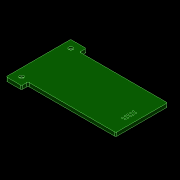
# Autodesk Inventor part: hw_DAA - PCB Peripherals
Saved by Autodesk Inventor 2018 (Build 220112000, 112)
## iProperties
Created: 2024-03-13
Part Number: hw_DAA - PCB Peripherals
Material: PCB
Document SubType Name: Modeling
Designer: cda1
Density: 4 g/cm^3
Appearance: PCB
Author: cda1
Autodesk Inventor part; units mm, degrees
ref_plane "YZ Plane" through (0, 0, 0) normal (1, 0, 0) x (0, 1, 0)
ref_plane "XZ Plane" through (0, 0, 0) normal (0, 1, 0) x (-1, 0, 0)
ref_plane "XY Plane" through (0, 0, 0) normal (0, 0, 1) x (1, 0, 0)
sketch "Boceto1" plane through (0, 0, 0) normal (0, 0, 1) x (1, 0, 0)
  line L0 (-26, 17) -> (26, 17)
  line L1 (26, 17) -> (26, -17)
  line L2 (26, -17) -> (-26, -17)
  line L3 (-26, -17) -> (-26, 17)
  line L4 (-26, 17) -> (26, -17) construction
  line L5 (26, 17) -> (-26, -17) construction
  point P0 (0, 0)
  dimension "d0" = 52
  dimension "d1" = 34
  constraints: 12 end point, 2 midpoint, 2 parallel, 1 horizontal, 1 perpendicular
  measures "d0" distance of L1.end L2.end
  measures "d1" distance of L0.end L1.end
extrude "Extrusión1" add sketch "Boceto1" against normal blind 1.742
fillet "Empalme1" radius 0.5 4 edges at (26, 17, -0.871) (-26, 17, -0.871) (-26, -17, -0.871) (26, -17, -0.871)
sketch "Boceto2" plane through (0, 0, -1.742) normal (0, 0, -1) x (-1, 0, 0)
  line L0 (-25.5, 17) -> (25.5, 17) projected
  line L1 (25.5, -17) -> (-25.5, -17) projected
  line L2 (25.5, 17) -> (-25.5, 17) projected
  line L3 (15.5, 17) -> (-26, 17)
  line L4 (-26, 17) -> (-26, 12.2)
  line L5 (-26, 12.2) -> (15.5, 12.2)
  line L6 (15.5, 12.2) -> (15.5, 17)
  line L7 (-26, -16.5) -> (-26, 16.5) projected
  line L8 (-25.5, -17) -> (25.5, -17) projected
  line L9 (-26, 16.5) -> (-26, -16.5) projected
  line L10 (15.5, -17) -> (-26, -17)
  line L11 (-26, -17) -> (-26, -12.2)
  line L12 (-26, -12.2) -> (15.5, -12.2)
  line L13 (15.5, -12.2) -> (15.5, -17)
  point P0 (0, 0)
  dimension "d5" = 4.8
  dimension "d6" = 41.5
  dimension "d7" = 4.8
  dimension "d8" = 41.5
  constraints: 16 end point, 4 parallel, 4 point on line, 2 horizontal, 2 perpendicular
  measures "d5" distance of L4.end L3.end
  measures "d6" distance of L4.end L5.end
  measures "d7" distance of L10.end L11.end
  measures "d8" distance of L11.end L12.end
extrude "Extrusión2" cut sketch "Boceto2" against normal through all
sketch "Boceto4" plane through (0, 0, 0) normal (0, 0, 1) x (1, 0, 0)
  line L0 (-26, -16.5) -> (-26, 16.5) construction
  line L1 (-26, 17) -> (-22.8, 17)
  line L2 (-22.8, 17) -> (-22.8, -17)
  line L3 (-22.8, -17) -> (-26, -17)
  line L4 (-26, -17) -> (-26, 17)
  line L5 (-15.5, -17) -> (-25.5, -17) projected
  line L6 (-25.5, 17) -> (-15.5, 17) projected
  point P0 (0, 0)
  dimension "d17" = 3.2
  constraints: 8 end point, 3 point on line, 2 parallel, 1 horizontal, 1 perpendicular
  measures "d17" distance of L2.end L3.end
extrude "Extrusión4" cut sketch "Boceto4" against normal up to surface (1.742 mm away)
sketch "Boceto7" plane through (0, 0, -1.742) normal (0, 0, -1) x (-1, 0, 0)
  line L0 (22.8, -17) -> (22.8, 17) projected
  line L1 (22.8, 17) -> (15.5, 17) projected
  line L2 (15.5, -17) -> (22.8, -17) projected
  point P0 (0, 0)
  point P1 (19.1, 11.638)
  point P2 (19.1, -11.638)
  dimension "d30" = 3.7
  dimension "d31" = 5.362
  dimension "d32" = 5.362
  constraints: 1 vertical alignment
  measures "d30" distance from line of L0 point (19.1, -11.638)
  measures "d31" distance from line of L1 point (19.1, 11.638)
  measures "d32" distance from line of L2 point (19.1, -11.638)
hole "Agujero2" at (-19.1, 11.638, -1.742) at (-19.1, -11.638, -1.742) direction (0, 0, 1) diameter 2 end through all countersink diameter 4 countersink angle 90
fillet "Empalme2" radius 0.5 8 edges at (-15.5, 17, -0.871) (-22.8, 17, -0.871) (-15.5, 12.2, -0.871) (26, 12.2, -0.871) (26, -12.2, -0.871) (-15.5, -12.2, -0.871) (-15.5, -17, -0.871) (-22.8, -17, -0.871)
sketch "Boceto8" plane through (0, 0, -1.742) normal (0, 0, -1) x (-1, 0, 0)
  line L0 (-26, 11.7) -> (-26, -11.7) construction
  line L1 (-25.5, -12.2) -> (15, -12.2) construction
  circle A0 centre (-22.735, 0.54) radius 0.37
  circle A1 centre (-21.465, 0.54) radius 0.37
  circle A2 centre (-22.735, -0.73) radius 0.37
  circle A3 centre (-21.465, -0.73) radius 0.37
  circle A4 centre (-22.735, -2) radius 0.37
  circle A5 centre (-21.465, -2) radius 0.37
  circle A6 centre (-22.735, -3.27) radius 0.37
  circle A7 centre (-21.465, -3.27) radius 0.37
  circle A8 centre (-22.735, -4.54) radius 0.37
  circle A9 centre (-21.465, -4.54) radius 0.37
  point P0 (0, 0)
  dimension "d49" = 3.265
  dimension "d50" = 1.27
  dimension "d51" = 1.27
  dimension "d52" = 1.27
  dimension "d53" = 1.27
  dimension "d54" = 12.74
  dimension "d55" = 0.74
  dimension "d56" = 0.74
  dimension "d57" = 0.74
  dimension "d58" = 0.74
  dimension "d59" = 0.74
  dimension "d60" = 0.74
  dimension "d61" = 0.74
  dimension "d62" = 0.74
  dimension "d63" = 1.27
  dimension "d64" = 0.74
  dimension "d65" = 0.74
  constraints: 10 centre point, 10 coincident, 8 vertical alignment, 5 horizontal alignment
  measures "d49" distance from line of L0 point (-22.735, 0.54)
  measures "d50" distance of point (-22.735, -0.73) point (-22.735, 0.54)
  measures "d51" distance of point (-22.735, -2) point (-22.735, -0.73)
  measures "d52" distance of point (-22.735, -3.27) point (-22.735, -2)
  measures "d53" distance of point (-22.735, 0.54) point (-21.465, 0.54)
  measures "d54" distance from line of L1 point (-22.735, 0.54)
  measures "d55" diameter of A0
  measures "d56" diameter of A1
  measures "d57" diameter of A2
  measures "d58" diameter of A3
  measures "d59" diameter of A4
  measures "d60" diameter of A5
  measures "d61" diameter of A6
  measures "d62" diameter of A7
  measures "d63" distance of A6.centre point (-22.735, -4.54)
  measures "d64" diameter of A8
  measures "d65" diameter of A9
extrude "Extrusión5" cut sketch "Boceto8" against normal up to surface (1.742 mm away)
sketch "Boceto9" plane through (0, 0, -1.742) normal (0, 0, -1) x (-1, 0, 0)
  line L0 (22.8, -17) -> (15.5, -17)
  line L1 (15.5, -17) -> (15.5, -15.258)
  line L2 (15.5, -15.258) -> (22.8, -15.258)
  line L3 (22.8, -15.258) -> (22.8, -17)
  line L4 (22.8, 15.258) -> (15.5, 15.258)
  line L5 (15.5, 15.258) -> (15.5, 17)
  line L6 (15.5, 17) -> (22.8, 17)
  line L7 (22.8, 17) -> (22.8, 15.258)
  point P0 (0, 0)
  point P1 (22.3, -17)
  point P2 (22.8, -16.5)
  point P3 (15.5, -16.5)
  point P4 (16, 17)
  point P5 (22.8, 16.5)
  point P6 (15.5, 16.5)
  dimension "d43" = 1.742
  dimension "d44" = 1.742
  constraints: 16 end point, 6 point on line, 4 parallel, 2 horizontal, 2 perpendicular
  measures "d43" distance of L0.end L1.end
  measures "d44" distance of L4.end L5.end
extrude "Extrusión6" cut sketch "Boceto9" against normal up to surface (1.742 mm away)
fillet "Empalme3" radius 0.5 4 edges at (-22.8, -15.258, -0.871) (-15.5, -15.258, -0.871) (-22.8, 15.258, -0.871) (-15.5, 15.258, -0.871)
